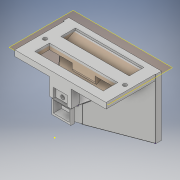
# Autodesk Inventor part: ventilador controladora
Saved by Autodesk Inventor 2019 (Build 230136000, 136)
## iProperties
Created: 2018-08-15
Part Number: ventilador controladora
Material: Genérico
Document SubType Name: Modeling
Designer: Albert Garangou Culebras
Density: 1 g/cm^3
Appearance: Valor por defecto
Author: Albert Garangou Culebras
Autodesk Inventor part; units mm, degrees
sketch "Boceto1" plane through (0, 0, 0) normal (0, 0, 1) x (1, 0, 0)
  line L0 (0, 0) -> (16, 0)
  line L1 (16, 0) -> (16, -12)
  line L2 (16, -12) -> (0, -12)
  line L3 (0, -12) -> (0, 0)
  line L4 (1, -1) -> (15, -1)
  line L5 (15, -1) -> (15, -11)
  line L6 (15, -11) -> (1, -11)
  line L7 (1, -11) -> (1, -1)
  dimension "d0" = 16
  dimension "d1" = 12
  constraints: 16 end point, 4 parallel, 2 horizontal, 2 perpendicular
  measures "d0" distance of L1.end L2.end
  measures "d1" distance of L0.end L1.end
ref_plane "Plano de trabajo3" through (0, 0, -40) normal (0, 0, -1) x (-1, 0, 0)
sketch "Boceto4" plane through (0, 0, -40) normal (0, 0, -1) x (-1, 0, 0)
  line L0 (0, -12) -> (0, 0) projected
  line L1 (0, -6) -> (-16, -6)
  line L2 (-8, -31) -> (-48, -31)
  line L3 (-8, -31) -> (32, -31)
  line L4 (32, -31) -> (32, 19)
  line L5 (32, 19) -> (-48, 19)
  line L6 (-48, 19) -> (-48, -31)
  dimension "d8" = 40
  dimension "d9" = 40
  dimension "d10" = 80
  constraints: 12 end point, 2 horizontal, 1 midpoint, 1 perpendicular, 1 vertical
  measures "d8" distance of L2.start L2.end
  measures "d9" distance of L2.start L3.end
  measures "d10" distance of L4.end L5.end
extrude "Extrusión2" add sketch "Boceto1" against normal blind 40
loft "Solevación1" add profiles "Boceto4" section 1 edges at (1, -6, 0) (8, -1, 0) (15, -6, 0) (8, -11, 0)
sketch "Boceto5" plane through (0, 0, -40) normal (0, 0, -1) x (-1, 0, 0)
  line L0 (30, -29) -> (-46, -29)
  line L1 (-46, -29) -> (-46, 17)
  line L2 (-46, 17) -> (30, 17)
  line L3 (30, 17) -> (30, -29)
  point P0 (0, 0)
  constraints: 8 end point, 2 parallel, 1 horizontal, 1 perpendicular
sketch "Boceto6" plane through (0, 0, 0) normal (0, 0, 1) x (1, 0, 0)
  line L0 (1, -11) -> (15, -11)
  line L1 (15, -11) -> (15, -1)
  line L2 (15, -1) -> (1, -1)
  line L3 (1, -1) -> (1, -11)
  point P0 (0, 0)
  constraints: 8 end point, 2 parallel, 1 horizontal, 1 perpendicular
loft "Solevación2" cut profiles "Boceto6", "Boceto5"
sketch "Boceto7" plane through (0, 0, 0) normal (0, 0, 1) x (1, 0, 0)
  line L0 (0, 0) -> (16, 0) projected
  line L1 (16, -12) -> (0, -12) projected
  line L2 (0, 0) -> (16, 0)
  line L3 (16, 0) -> (16, -12)
  line L4 (16, -12) -> (0, -12)
  line L5 (0, -12) -> (0, 0)
  line L6 (1, -11) -> (1, -1) projected
  line L7 (1, -1) -> (15, -1)
  line L8 (15, -1) -> (15, -11)
  line L9 (15, -11) -> (1, -11)
  line L10 (1, -11) -> (1, -1)
  constraints: 16 end point, 4 parallel, 2 horizontal, 2 perpendicular
extrude "Extrusión3" add sketch "Boceto7" against normal blind 5
sketch "Boceto8" plane through (0, 0, 0) normal (0, 0, 1) x (1, 0, 0)
  line L0 (0, 0) -> (16, 0)
  line L1 (16, 0) -> (16, -12)
  line L2 (16, -12) -> (0, -12)
  line L3 (0, -12) -> (0, 0)
  line L4 (15, -1) -> (15, -11) projected
  line L5 (1, -1) -> (15, -1)
  line L6 (15, -1) -> (15, -11)
  line L7 (15, -11) -> (1, -11)
  line L8 (1, -11) -> (1, -1)
  constraints: 16 end point, 4 parallel, 2 horizontal, 2 perpendicular
extrude "Extrusión4" add sketch "Boceto8" along normal blind 3
ref_plane "Plano de trabajo7" through (-19.527001, -29, -48.116575) normal (0.7904151, 0, -0.6125717) x (-0.6125717, 0, -0.7904151)
sketch "Boceto17" plane through (-19.527001, -29, -48.116575) normal (0.7904151, 0, -0.6125717) x (-0.6125717, 0, -0.7904151)
  line L0 (-46.555447, 46) -> (0, 46)
  line L1 (-10.291798, 46) -> (-10.291798, 0)
  line L2 (-10.291798, 0) -> (-38.576069, 10)
  line L3 (-38.576069, 10) -> (-38, 37)
  line L4 (-38, 37) -> (-10.291798, 46)
  point P0 (-49.993752, 29)
  dimension "d37" = 30
  constraints: 8 end point, 1 point on line, 1 vertical
  measures "d37" distance of L1.end L2.end
ref_plane "Plano de trabajo8" through (35.724604, -29, -47.963432) normal (-0.7904151, 0, -0.6125717) x (-0.6125717, 0, 0.7904151)
sketch "Boceto18" plane through (35.724604, -29, -47.963432) normal (-0.7904151, 0, -0.6125717) x (-0.6125717, 0, 0.7904151)
  line L0 (0, 46) -> (46.555447, 46)
  line L1 (10.079184, 46) -> (10.079184, 0)
  line L2 (46.555447, 0) -> (0, 0)
  line L3 (10.079184, 0) -> (38.363455, 10)
  line L4 (38.363455, 10) -> (38.363455, 36)
  line L5 (38.363455, 36) -> (10.079184, 46)
  point P0 (59.794899, 29)
  dimension "d39" = 30
  constraints: 8 end point, 2 point on line, 2 vertical
  measures "d39" distance of L1.end L3.end
extrude "Extrusión9" add sketch "Boceto18" along normal blind 0.8
extrude "Extrusión10" add sketch "Boceto17" along normal blind 0.8
ref_plane "Plano de trabajo9" through (0, 19, -2) normal (0, 1, 0) x (1, 0, 0)
sketch "Boceto22" plane through (0, 19, -2) normal (0, 1, 0) x (1, 0, 0)
  line L0 (-13.199031, 38) -> (-30, 38)
  line L1 (-30, 38) -> (13, 38) construction
  line L2 (16, -0.787879) -> (48, 38)
  line L3 (48, 38) -> (48, -5)
  line L4 (48, 38) -> (91, 38) construction
  line L5 (48, -5) -> (-31.751276, -5)
  line L6 (48, 38) -> (-32, 38)
  line L7 (-31.751276, 38) -> (-31.751276, -5)
  line L8 (-31.751276, 38) -> (11.248724, 38) construction
  line L9 (-31.751276, -5) -> (-21.751276, -5)
  line L10 (-21.751276, -5) -> (-21.751276, 38)
  line L11 (-21.751276, 38) -> (-31.751276, 38)
  line L12 (48, -5) -> (38, -5)
  line L13 (38, -5) -> (38, 38)
  line L14 (48, 38) -> (38, 38)
  point P0 (0, -2)
  dimension "d46" = 90
  dimension "d47" = 43
  dimension "d49" = 90
  dimension "d50" = 10
  dimension "d51" = 43
  dimension "d52" = 90
  dimension "d53" = 10
  dimension "d54" = 43
  constraints: 24 end point, 4 perpendicular, 4 point on line, 3 horizontal, 1 collinear
  measures "d46" angle of L3 L4
  measures "d47" distance of L2.end L3.end
  measures "d49" angle of L7 L8
  measures "d50" distance of L5.end L9.end
  measures "d51" distance of L9.end L10.end
  measures "d52" angle of L10 L9
  measures "d53" distance of L3.end L12.end
  measures "d54" distance of L12.end L13.end
extrude "Extrusión11" add sketch "Boceto22" against normal blind 3 contours L10 L5 L7 L6 L0 | L6 L2 L13 | L3 L5 L13 L2
sketch "Boceto24" plane through (38, 19, -40) normal (-1, 0, 0) x (0, 0, 1)
  line L0 (0, 0) -> (43, 0) projected
  line L1 (35.5, -2) -> (35.5, 0)
  line L2 (35.5, 0) -> (43, 0)
  line L3 (43, 0) -> (43, -2)
  line L4 (35.5, -2) -> (35.5, -3)
  line L5 (43, -3) -> (6, -3) projected
  line L6 (43, -3) -> (35.5, -3)
  line L7 (43, -3) -> (43, -2)
  line L8 (43, 0) -> (43, -3) projected
  point P0 (40, -19)
  dimension "d57" = 7.5
  constraints: 12 end point, 2 collinear, 2 point on line, 1 parallel, 1 vertical
  measures "d57" distance of L1.end L2.end
extrude "Extrusión12" add sketch "Boceto24" along normal blind 60
sketch "Boceto25" plane through (-31.751276, 19, 3) normal (0, 0, 1) x (1, 0, 0)
  line L0 (79.751276, -3) -> (0, -3)
  line L1 (39.875638, -3) -> (49.375638, -3)
  line L2 (39.875638, -3) -> (30.375638, -3)
  line L3 (30.375638, -3) -> (30.375638, -19)
  line L4 (30.375638, -19) -> (49.375638, -19)
  line L5 (49.375638, -19) -> (49.375638, -3)
  point P0 (31.751276, -19)
  dimension "d60" = 9.5
  dimension "d61" = 9.5
  dimension "d63" = 16
  dimension "d64" = 19
  constraints: 10 end point, 2 perpendicular, 2 point on line, 1 midpoint
  measures "d60" distance of L1.start L1.end
  measures "d61" distance of L1.start L2.end
  measures "d63" distance of L2.end L3.end
  measures "d64" distance of L3.end L4.end
extrude "Extrusión13" add sketch "Boceto25" against normal blind 7.5
sketch "Boceto27" plane through (0, 0, -40) normal (0, 0, -1) x (-1, 0, 0)
  line L0 (31.751276, 19) -> (-48, 19)
  line L1 (31.751276, 19) -> (-48, 19)
  line L2 (-48, 19) -> (-48, -31)
  line L3 (-48, -31) -> (31.751276, -31)
  line L4 (31.751276, -31) -> (31.751276, 19)
  line L5 (30, 16) -> (30, -29)
  line L6 (-46, -29) -> (-46, 16)
  line L7 (30, 17) -> (-46, 17)
  line L8 (-46, 17) -> (-46, -29)
  line L9 (-46, -29) -> (30, -29)
  line L10 (30, -29) -> (30, 17)
  point P0 (0, 0)
  constraints: 16 end point, 4 parallel, 2 horizontal, 2 perpendicular
extrude "Extrusión15" add sketch "Boceto27" along normal blind 5
sketch "Boceto28" plane through (0, -12, -2) normal (0, -1, 0) x (1, 0, 0)
  line L0 (16, 1) -> (0, 1)
  line L1 (0, 1) -> (0, 5)
  line L2 (0, 5) -> (16, 5)
  line L3 (16, 5) -> (16, 1)
  point P0 (0, 2)
  constraints: 8 end point, 2 parallel, 1 horizontal, 1 perpendicular
extrude "Extrusión16" add sketch "Boceto28" against normal blind 12
sketch "Boceto30" plane through (0, 0, 3) normal (0, 0, 1) x (1, 0, 0)
  line L0 (15, -11) -> (1, -11)
  line L1 (1, -11) -> (1, -1)
  line L2 (1, -1) -> (15, -1)
  line L3 (15, -1) -> (15, -11)
  point P0 (0, 0)
  constraints: 8 end point, 2 parallel, 1 horizontal, 1 perpendicular
extrude "Extrusión17" cut sketch "Boceto30" against normal blind 7.75
sketch "Boceto31" plane through (-32, -31, -40) normal (-0.7713733, 0, 0.636383) x (0.636383, 0, 0.7713733)
  line L0 (50.223865, 30.580645) -> (50.223865, 19.419355)
  line L1 (50.223865, 30.580645) -> (50.223865, 19.419355)
  line L2 (50.223865, 19.419355) -> (36, 14)
  line L3 (36, 14) -> (36, 36.115281)
  line L4 (50.284188, 30.606061) -> (7.778335, 47)
  line L5 (50.223865, 30.580645) -> (36, 36.115281)
  point P0 (51.219186, 31)
  constraints: 8 end point, 1 collinear, 1 parallel, 1 point on line
extrude "Extrusión18" add sketch "Boceto31" against normal blind 1
sketch "Boceto32" plane through (16, -11.606061, -1.212121) normal (0.7713733, 0, 0.636383) x (0.636383, 0, -0.7713733)
  line L0 (0.060322, 11.186706) -> (0.779165, 11.606061)
  line L1 (0.060322, -0.000081) -> (0.060322, 11.186706)
  line L2 (0.060322, 11.186706) -> (9.130626, 14.733682)
  line L3 (0, 11.212121) -> (42.505852, 27.606061)
  line L4 (9.130626, -0.000163) -> (9.130626, 14.733682)
  line L5 (-0.626449, 30.606061) -> (-0.626449, -19.393939)
  line L6 (9.130626, -0.000163) -> (9.130626, -3.535488)
  line L7 (9.130626, -3.535488) -> (0.060322, -0.000325)
  line L8 (0.060322, 0.025415) -> (0.060322, 11.186706)
  line L9 (0.060322, -0.000325) -> (0.060322, 11.186706)
  point P0 (-11.117125, 11.606061)
  constraints: 12 end point, 2 vertical, 1 collinear, 1 parallel, 1 point on line
extrude "Extrusión19" add sketch "Boceto32" against normal blind 1 contours L2 L4 L6 L7 L1
sketch "Boceto33" plane through (0, -12, -2) normal (0, -0.8944272, 0.4472136) x (1, 0, 0)
  line L0 (0, -0.700786) -> (0, 4.665778)
  line L1 (0, 0.854238) -> (-9.541728, -11.818024)
  line L2 (-8.31884, -11.8619) -> (-4.377414, -6.627335)
  line L3 (-9.541728, -11.818024) -> (25.370549, -11.818024)
  line L4 (11.591907, -17.557996) -> (11.591907, -5.930443)
  line L5 (16, 0.880875) -> (19.630054, -4.038548)
  line L6 (25.370549, -11.818024) -> (16, 0.880875)
  line L7 (16, 4.472136) -> (16, 0)
  line L8 (16, 0.880875) -> (16, 0)
  line L9 (16, 0) -> (0, 0)
  line L10 (0, 0) -> (0, 0.854238)
  line L11 (0, 4.472136) -> (0, 0)
  point P0 (0, 7.155418)
  point P1 (0, 0.09651)
  point P2 (0, 5.275946)
  constraints: 12 end point, 3 point on line, 2 collinear, 1 parallel, 1 perpendicular
extrude "Extrusión20" add sketch "Boceto33" against normal blind 1
sketch "Boceto34" plane through (0, 0, -2) normal (0, 0.8944272, 0.4472136) x (1, 0, 0)
  line L0 (30.35, 18.56614) -> (-13.525, 17.448106)
  line L1 (0, -0.880875) -> (-27.05, 35.777088)
  line L2 (-13.525, 17.448106) -> (0.825, -1.998909)
  line L3 (0.825, -1.998909) -> (0, -0.036399)
  line L4 (0, 0) -> (0, -0.880875)
  line L5 (0, 0) -> (16, 0)
  line L6 (16, 0) -> (0, 0)
  line L7 (16, -0.880875) -> (16, 0)
  line L8 (16, 0) -> (16, -0.880875)
  line L9 (16, -0.880875) -> (30.35, 18.56614)
  line L10 (16, -0.880875) -> (43.05, 35.777088)
  point P0 (0, -1.788854)
  point P1 (17.624362, 2.236068)
  point P2 (17.624362, 2.795085)
  constraints: 12 end point, 2 collinear, 1 midpoint, 2 other
extrude "Extrusión21" [suppressed]
sketch "Boceto35" plane through (16, -11.606061, -1.212121) normal (0.7713733, 0, 0.636383) x (0.636383, 0, -0.7713733)
  line L0 (0, 0) -> (16, -6.170986)
  line L1 (9.130626, -3.52156) -> (50.284188, -19.393939)
  line L2 (16, -6.170986) -> (16, 17.383107)
  line L3 (0, 11.212121) -> (42.505852, 27.606061)
  line L4 (0, 0) -> (0, 11.212121)
  line L5 (0, 11.212121) -> (16, 17.383107)
  line L6 (0, 11.212121) -> (0.607749, 11.606061)
  line L7 (0, 11.212121) -> (0, 0)
  line L8 (1.212121, 11.606061) -> (1.212121, 0.332344)
  point P0 (-11.117125, 11.606061)
  point P1 (1.212121, 10.879778)
  point P2 (1.212121, 0.332344)
  point P3 (0.30303, 10.426431)
  point P4 (0.30303, 0.78569)
  constraints: 8 end point, 2 point on line, 2 vertical, 1 other
extrude "Extrusión22" add sketch "Boceto35" against normal blind 1
sketch "Boceto37" plane through (0, 0, 3) normal (0, 0, 1) x (1, 0, 0)
  line L0 (0, -12) -> (16, -12) projected
  line L1 (0, -12) -> (16, -12)
  line L2 (16, -12) -> (16, 0)
  line L3 (16, 0) -> (0, 0)
  line L4 (0, 0) -> (0, -12)
  line L5 (1, -1) -> (15, -1) projected
  line L6 (15, -1) -> (1, -1)
  line L7 (1, -1) -> (1, -11)
  line L8 (1, -11) -> (15, -11)
  line L9 (15, -11) -> (15, -1)
  constraints: 16 end point, 4 parallel, 2 horizontal, 2 perpendicular
extrude "Extrusión23" cut sketch "Boceto37" against normal blind 1
sketch "Boceto38" plane through (-31.751276, 19, 3) normal (0, 0, 1) x (1, 0, 0)
  line L0 (30.375638, -17.75) -> (49.375638, -17.75)
  line L1 (30.375638, -19) -> (49.375638, -19)
  line L2 (39.875638, -19) -> (39.875638, -14)
  line L3 (39.875638, -14) -> (39.875638, -15)
  circle A0 centre (39.875638, -15) radius 1.75
  point P0 (31.751276, -19)
  dimension "d94" = 5
  dimension "d146" = 1
  dimension "d147" = 3.5
  constraints: 4 end point, 2 coincident, 1 centre point, 1 midpoint, 1 point on line
  measures "d94" distance of L2.start L2.end
  measures "d146" distance of L3.start L3.end
  measures "d147" diameter of A0
extrude "Extrusión24" cut sketch "Boceto38" against normal blind 7.75
sketch "Boceto39" plane through (-31.751276, 19, 3) normal (0, 0, 1) x (1, 0, 0)
  line L0 (34.424818, -19) -> (45.424818, -19)
  line L1 (45.424818, -9.5) -> (45.674818, -9.5)
  line L2 (45.674818, -9.5) -> (45.674818, -19)
  line L3 (16.800456, -9.5) -> (16.550456, -9.5)
  line L4 (45.674818, -19) -> (33.674818, -19)
  line L5 (45.424818, -9.5) -> (33.674818, -9.5)
  line L6 (33.674818, -19) -> (33.674818, -9.5)
  line L7 (30.375638, -17.75) -> (49.375638, -17.75)
  point P0 (30.375638, -3)
  point P1 (49.375638, -3)
  point P2 (16.550456, -19)
  dimension "d100" = 9.5
  dimension "d103" = 0.25
  dimension "d104" = 0.25
  dimension "d109" = 12
  constraints: 14 end point, 2 perpendicular, 1 horizontal
  measures "d100" distance of L0.end L1.start
  measures "d103" distance of L1.start L1.end
  measures "d104" distance of L3.start L3.end
  measures "d109" distance of L2.end L4.end
extrude "Extrusión25" cut sketch "Boceto39" against normal blind 2
sketch "Boceto40" plane through (0, 16, -2) normal (0, -1, 0) x (1, 0, 0)
  line L0 (-31.751276, -38) -> (-31.751276, 5)
  line L1 (-31.751276, 5) -> (-31.751276, -38)
  line L2 (-31.751276, -16.5) -> (-22, -16.5)
  circle A0 centre (-26.875638, -16.5) radius 1.65
  circle A1 centre (43, -16.5) radius 1.65
  point P0 (0, 2)
  dimension "d105" = 3.3
  dimension "d106" = 3.3
  constraints: 4 end point, 2 centre point, 2 midpoint, 1 collinear, 1 horizontal
  measures "d105" diameter of A0
  measures "d106" diameter of A1
extrude "Extrusión26" cut sketch "Boceto40" against normal blind 38.5
sketch "Boceto41" plane through (0, 16, -2) normal (0, -1, 0) x (1, 0, 0)
  line L0 (38, -35.777778) -> (38, -38)
  line L1 (38, -35.777778) -> (38, -38)
  line L2 (38, -38) -> (46, -38)
  line L3 (38, -38) -> (46, -38)
  line L4 (46, -38) -> (44.288464, -35.777778)
  line L5 (44.288464, -35.777778) -> (38, -35.777778)
  line L6 (-21.751276, -2.5) -> (-21.751276, -38)
  line L7 (-21.751276, -35.777778) -> (-21.751276, -38)
  line L8 (-30, -38) -> (-21.751276, -38)
  line L9 (-21.751276, -38) -> (-30, -38)
  line L10 (-30, -38) -> (-28.277778, -35.777778)
  line L11 (-30, -38) -> (-28.277778, -35.777778)
  line L12 (-28.277778, -35.777778) -> (-21.751276, -35.777778)
  line L13 (-28.277778, -35.777778) -> (-21.751276, -35.777778)
  point P0 (0, 2)
  constraints: 16 end point, 4 collinear, 2 parallel, 1 perpendicular, 1 point on line
extrude "Extrusión27" cut sketch "Boceto41" against normal blind 1
sketch "Boceto42" plane through (38, 16, -37.777778) normal (1, 0, 0) x (0, 0, -1)
  line L0 (2.222222, 1) -> (0, 1)
  line L1 (0, 0) -> (0, 1)
  line L2 (2.222222, 1) -> (0, 0)
  line L3 (0, 0) -> (0, 1)
  line L4 (0, 1) -> (2.222222, 1)
  point P0 (-37.777778, -16)
  constraints: 6 end point, 1 collinear, 1 perpendicular
sketch "Boceto43" plane through (-21.751276, 16, -37.777778) normal (-1, 0, 0) x (0, 0, 1)
  line L0 (0, 0) -> (-2.222222, 1)
  line L1 (-2.222222, 1) -> (0, 0)
  line L2 (0, 0) -> (0, 1)
  line L3 (0, 0) -> (0, 1)
  line L4 (0, 1) -> (-2.222222, 1)
  point P0 (37.777778, -16)
  constraints: 6 end point, 2 collinear, 1 perpendicular
extrude "Extrusión29" add sketch "Boceto43" along normal blind 8.75
extrude "Extrusión30" add sketch "Boceto42" along normal blind 8.25
sketch "Boceto44" plane through (0, 0, 3) normal (0, 0, 1) x (1, 0, 0)
  line L0 (13.923542, 0) -> (17.624362, 0)
  line L1 (17.624362, 0) -> (17.624362, 1)
  line L2 (17.624362, 1.25) -> (17.624362, 0.590523)
  line L3 (17.624362, 1.025) -> (-1.375638, 1.025)
  line L4 (17.624362, 1) -> (-1.375638, 1.025)
  line L5 (-1.375638, 1.025) -> (-1.376954, 0.025002)
  line L6 (-1.376954, 0.025002) -> (17.624362, 0)
  point P0 (0, 0)
  dimension "d118" = 1
  constraints: 8 end point, 2 perpendicular, 1 point on line
  measures "d118" distance of L0.end L1.end
extrude "Extrusión31" cut sketch "Boceto44" against normal blind 7.25 contours L6 L5 L4 L1
sketch "Boceto45" plane through (-0.65, 0, -2) normal (0, -1, 0) x (1, 0, 0)
  line L0 (-0.725638, 5) -> (2.573542, 5)
  line L1 (2.573542, 5) -> (-0.725638, 5)
  line L2 (-0.725638, 5) -> (-0.725638, -0.879561)
  line L3 (-0.725638, 5) -> (-0.725638, -0.879561)
  line L4 (0.65, 0) -> (0.65, 0.787879)
  line L5 (-0.725638, -0.879561) -> (0.65, 0)
  line L6 (0.65, 0) -> (0.65, 4)
  line L7 (0.65, 4) -> (2.573542, 4)
  line L8 (2.573542, 4) -> (2.573542, 5)
  line L9 (2.573542, 4) -> (2.573542, 5)
  line L10 (14.573542, 5) -> (18.274362, 5)
  line L11 (14.573542, 5) -> (18.274362, 5)
  line L12 (18.274362, 5) -> (14.573542, 5)
  line L13 (2.573542, 4) -> (14.573542, 4)
  line L14 (14.573542, 5) -> (14.573542, 4)
  line L15 (14.573542, 4) -> (16.65, 4)
  line L16 (16.65, 0.787879) -> (16.65, 0)
  line L17 (16.65, 4) -> (16.65, 0.787879)
  line L18 (18.274362, -1.181045) -> (17.3, 0)
  line L19 (16.65, 0.787879) -> (18.274362, -1.181045)
  line L20 (18.274362, 5) -> (18.274362, -1.181045)
  line L21 (18.274362, -1.181045) -> (18.274362, 5)
  line L22 (18.274362, 5) -> (14.573542, 5)
  point P0 (0.65, 2)
  constraints: 26 end point, 7 perpendicular, 3 collinear, 1 horizontal, 1 parallel
extrude "Extrusión32" cut sketch "Boceto45" against normal blind 0.5
sketch "Boceto46" plane through (-21.751276, 19, -4.5) normal (1, 0, 0) x (0, 0, -1)
  line L0 (35.5, 0) -> (29.5, -3)
  line L1 (0, 0) -> (35.5, 0)
  line L2 (35.5, 0) -> (0, 0)
  line L3 (17.75, 0) -> (22.75, 0)
  line L4 (22.75, 0) -> (12.75, 0)
  line L5 (22.75, 0) -> (22.75, -3)
  line L6 (-7.5, -3) -> (35.198516, -3)
  line L7 (22.75, -3) -> (12.75, -3)
  line L8 (15.65, -3) -> (12.35, -3)
  line L9 (29.5, -3) -> (0, -3)
  line L10 (12.75, -3) -> (12.75, 0)
  point P0 (-4.5, -19)
  dimension "d123" = 5
  dimension "d124" = 10
  constraints: 12 end point, 4 point on line, 1 collinear, 1 midpoint, 1 perpendicular, 1 vertical
  measures "d123" distance of L3.start L3.end
  measures "d124" distance of L3.end L4.end
extrude "Extrusión33" add sketch "Boceto46" along normal blind 61.5 contours L5 L6 L10 L1
sketch "Boceto47" plane through (0, 16, -2) normal (0, -1, 0) x (1, 0, 0)
  line L0 (38, -15.25) -> (38, -2.5)
  line L1 (-21.751276, -15.25) -> (38, -15.25)
  line L2 (38, -15.25) -> (-21.751276, -15.25)
  line L3 (-21.751276, -32) -> (-21.751276, -25.25)
  line L4 (-21.751276, -15.25) -> (-21.751276, -25.25)
  line L5 (-21.751276, -25.25) -> (38, -25.25)
  line L6 (-21.751276, -25.25) -> (38, -25.25)
  line L7 (38, -25.25) -> (38, -15.25)
  line L8 (-21.751276, -15.25) -> (-21.751276, -2.5)
  line L9 (-21.751276, -15.25) -> (-21.751276, -25.25)
  line L10 (8.124362, -15.25) -> (-1.875638, -15.25)
  line L11 (-1.875638, -15.25) -> (18.124362, -15.25)
  line L12 (18.124362, -15.25) -> (18.124362, -25.25)
  line L13 (-1.875638, -15.25) -> (-1.875638, -25.25)
  line L14 (18.124362, -25.25) -> (-1.875638, -25.25)
  point P0 (0, 2)
  dimension "d127" = 10
  dimension "d128" = 20
  constraints: 20 end point, 5 perpendicular, 4 point on line, 3 collinear, 1 midpoint
  measures "d127" distance of L10.start L10.end
  measures "d128" distance of L10.end L11.end
extrude "Extrusión34" add sketch "Boceto47" along normal blind 4.5 contours L1 L12 L5 L13
sketch "Boceto48" plane through (-21.751276, 19, -40) normal (0, 0.8944272, 0.4472136) x (1, 0, 0)
  line L0 (19.875638, -23.702321) -> (19.875638, -16.77051)
  line L1 (19.875638, -23.702321) -> (39.875638, -23.702321)
  line L2 (39.875638, -23.702321) -> (39.875638, -14.702321)
  line L3 (39.875638, -14.702321) -> (19.875638, -14.702321)
  line L4 (19.875638, -16.77051) -> (19.875638, -14.254933)
  line L5 (39.875638, -14.702321) -> (19.875638, -14.702321)
  point P0 (21.751276, -44.274146)
  dimension "d131" = 9
  constraints: 8 end point, 2 perpendicular, 1 collinear, 1 horizontal, 1 point on line
  measures "d131" distance of L1.end L2.end
extrude "Extrusión35" add sketch "Boceto48" along normal blind 7.25
sketch "Boceto49" plane through (0, 16, -2) normal (0, -1, 0) x (1, 0, 0)
  line L0 (-21.751276, -15.25) -> (-21.751276, -2.5)
  line L1 (-21.751276, -15.25) -> (-21.751276, -2.5)
  line L2 (38, -2.5) -> (17.624362, -2.5)
  line L3 (-21.751276, -2.5) -> (38, -2.5)
  line L4 (38, -2.5) -> (38, -15.25)
  line L5 (38, -2.5) -> (38, -15.25)
  line L6 (-21.751276, -15.25) -> (-1.875638, -15.25)
  line L7 (38, -15.25) -> (-21.751276, -15.25)
  point P0 (0, 2)
  constraints: 8 end point, 2 collinear, 1 perpendicular
extrude "Extrusión36" cut sketch "Boceto49" along normal blind 5.25
sketch "Boceto50" plane through (0, 19, -2) normal (0, 1, 0) x (1, 0, 0)
  line L0 (48, -5) -> (48, 43)
  line L1 (-31.751276, 43) -> (48, 43)
  line L2 (48, -5) -> (-31.751276, -5)
  line L3 (-31.751276, -5) -> (-31.751276, 43)
  line L4 (-31.751276, 43) -> (48, 43)
  line L5 (48, 43) -> (48, -5)
  line L6 (38, 2.5) -> (38, 15.25)
  line L7 (-21.751276, 15.25) -> (-21.751276, 2.5)
  line L8 (38, 2.5) -> (-21.751276, 2.5)
  line L9 (-21.751276, 2.5) -> (-21.751276, 15.25)
  line L10 (-21.751276, 15.25) -> (38, 15.25)
  line L11 (38, 15.25) -> (38, 2.5)
  line L12 (18.124362, 25.25) -> (38, 25.25)
  line L13 (-21.751276, 25.25) -> (-21.751276, 38)
  line L14 (38, 25.25) -> (-21.751276, 25.25)
  line L15 (-21.751276, 25.25) -> (-21.751276, 38)
  line L16 (-21.751276, 38) -> (38, 38)
  line L17 (38, 38) -> (38, 25.25)
  circle A0 centre (43, 16.5) radius 1.65
  circle A1 centre (43, 16.5) radius 1.65
  circle A2 centre (-26.875638, 16.5) radius 1.65
  circle A3 centre (-26.875638, 16.5) radius 1.65
  point P0 (0, -2)
  constraints: 24 end point, 6 parallel, 3 horizontal, 3 perpendicular, 2 centre point, 2 coincident
extrude "Extrusión37" add sketch "Boceto50" along normal blind 2
sketch "Boceto51" plane through (0, 0, 2) normal (0, 0, 1) x (1, 0, 0)
  line L0 (15, -0.488405) -> (0, -0.488405)
  line L1 (0, -0.488405) -> (0, 0.453578)
  line L2 (0, -12) -> (0, 0.02319)
  line L3 (0, 0.453578) -> (16.256322, 0.453578)
  line L4 (16.256322, 0.453578) -> (16.256322, -0.488405)
  line L5 (16.256322, -0.488405) -> (15, -0.488405)
  point P0 (0, 0)
  point P1 (0, -0.419355)
  point P2 (16, 0)
  point P3 (16, -0.393939)
  constraints: 10 end point, 2 collinear, 2 perpendicular, 1 horizontal, 1 point on line
extrude "Extrusión38" cut sketch "Boceto51" against normal blind 3.25
sketch "Boceto52" plane through (16, -12, 2) normal (1, 0, 0) x (0, 0, -1)
  line L0 (0, 0) -> (0, 11.511595)
  line L1 (0, 0) -> (0, 11.511595)
  line L2 (3.212121, 11.511595) -> (0, 11.511595)
  line L3 (0, 11.511595) -> (3.212121, 11.511595)
  line L4 (3.212121, 11.511595) -> (3.212121, 0)
  line L5 (3.212121, 11.511595) -> (3.212121, 0.393939)
  line L6 (0, 0) -> (4, 0)
  line L7 (3.212121, 0) -> (0, 0)
  point P0 (2, 12)
  constraints: 8 end point, 3 collinear, 1 vertical
extrude "Extrusión39" add sketch "Boceto52" along normal blind 0.3
sketch "Boceto53" plane through (0, -12, -2) normal (-1, 0, 0) x (0, 0, 1)
  line L0 (4, 11.511595) -> (0.787879, 11.511595)
  line L1 (4, 11.511595) -> (0.787879, 11.511595)
  line L2 (0.787879, 11.511595) -> (0.787879, 0)
  line L3 (4, 0) -> (0, 0)
  line L4 (0.787879, 0) -> (4, 0)
  line L5 (4, 0) -> (4, 11.511595)
  point P0 (2, 12)
  constraints: 8 end point, 2 collinear, 2 perpendicular
extrude "Extrusión40" add sketch "Boceto53" along normal blind 0.3
sketch "Boceto54" plane through (0, -12, -2) normal (0, -1, 0) x (1, 0, 0)
  line L0 (16, 0.787879) -> (16.3, 0.787879)
  line L1 (16.3, 4) -> (16.3, 0.787879)
  line L2 (16.3, 0.787879) -> (16.3, 4)
  line L3 (16.3, 4) -> (-0.3, 4)
  line L4 (16.3, 4) -> (-0.3, 4)
  line L5 (-0.3, 0.787879) -> (-0.3, 4)
  line L6 (-0.3, 4) -> (-0.3, 0.787879)
  line L7 (-0.3, 0.787879) -> (16.3, 0.787879)
  point P0 (0, 2)
  constraints: 8 end point, 2 collinear, 2 perpendicular
extrude "Extrusión41" add sketch "Boceto54" along normal blind 0.75
sketch "Boceto55" plane through (48, -31, -40) normal (0.7713733, 0, 0.636383) x (0.636383, 0, -0.7713733)
  line L0 (0, 0) -> (0, 47)
  line L1 (0, 47) -> (0, 0)
  line L2 (-49.676439, 19) -> (-50.284188, 19.393939)
  line L3 (0, 0) -> (-50.284188, 19.393939)
  line L4 (-47.731696, 31.590523) -> (-7.778335, 47)
  line L5 (-50.284188, 30.511595) -> (-7.778335, 47)
  line L6 (-7.778335, 47) -> (0, 47)
  line L7 (-1.272766, 48) -> (2.5841, 48)
  line L8 (-50.284188, 19.393939) -> (-44.57999, 17.193907)
  line L9 (-50.284188, 19.393939) -> (-45.619136, 17.594691)
  line L10 (-45.619136, 17.594691) -> (-45.08732, 17.389577)
  line L11 (-45.08732, 17.389577) -> (-45.08732, 32.527507)
  point P0 (-61.401313, 31)
  point P1 (-45.619136, 32.321211)
  dimension "d159" = 5
  dimension "d160" = 0.57
  constraints: 14 end point, 4 point on line, 1 collinear, 1 parallel, 1 vertical
  measures "d159" distance of L2.end L9.end
  measures "d160" distance of L9.end L10.end
extrude "Extrusión42" add sketch "Boceto55" along normal blind 0.4
sketch "Boceto56" plane through (-32, -31, -40) normal (-0.7713733, 0, 0.636383) x (0.636383, 0, 0.7713733)
  line L0 (50.284188, 19.393939) -> (49.676439, 19)
  line L1 (50.093273, 30.511595) -> (8.041918, 47)
  line L2 (7.778335, 47) -> (0.390841, 47)
  line L3 (8.041918, 47) -> (0.390841, 47)
  line L4 (0.390841, 47) -> (0.390841, 50)
  line L5 (0.390841, 49.849258) -> (0, 50)
  line L6 (0.390841, 50) -> (0, 50)
  line L7 (35.559487, 13.714819) -> (0, 0)
  line L8 (0, 50) -> (0, 0)
  line L9 (0, 0) -> (50.284188, 19.393939)
  line L10 (60.456983, 30.511595) -> (50.254969, 30.511595)
  line L11 (50.093273, 30.511595) -> (45.43832, 32.33681)
  line L12 (45.43832, 17.524953) -> (45.201514, 17.444807)
  line L13 (48.73986, 18.798313) -> (35.450552, 13.714819)
  line L14 (45.201514, 17.444807) -> (44.968015, 17.355487)
  line L15 (44.968015, 17.355487) -> (45.108115, 17.409079)
  line L16 (45.108115, 17.409079) -> (45.108115, 32.466284)
  point P0 (51.219186, 31)
  point P1 (59.443155, 30.511595)
  point P2 (45.201514, 32.429661)
  dimension "d155" = 5
  dimension "d156" = 0.25
  dimension "d157" = 0.25
  dimension "d158" = 0.15
  constraints: 22 end point, 10 point on line, 3 perpendicular, 1 collinear, 1 vertical
  measures "d155" distance of L11.start L11.end
  measures "d156" distance of L12.start L12.end
  measures "d157" distance of L12.end L14.end
  measures "d158" distance of L14.end L15.end
extrude "Extrusión43" add sketch "Boceto56" along normal blind 0.4 contours L16 L13 L12 L9 L7 L8 L5 L4 L2 L3 L1
sketch "Boceto57" plane through (0, -12, -2) normal (0, -0.8944272, 0.4472136) x (1, 0, 0)
  line L0 (-31.751276, -42.485292) -> (48, -42.485292)
  line L1 (-31.751276, -42.485292) -> (-31.751276, -46.957428)
  line L2 (48, -42.485292) -> (-31.751276, -42.485292)
  line L3 (-31.751276, -42.485292) -> (-32, -42.485292)
  line L4 (-32, -42.485292) -> (-32.308549, -42.257612)
  line L5 (-32, -42.485292) -> (-1.387902, -1)
  line L6 (-3.083828, -3.298306) -> (-32, -42.485292)
  line L7 (-0.340004, 0.420104) -> (-3.308764, -3.603137)
  line L8 (-3.308764, -3.603137) -> (19.308764, -3.603137)
  line L9 (19.307198, -3.601015) -> (19.630054, -4.038548)
  line L10 (48, -42.485292) -> (48, -21.466253)
  line L11 (19.308764, -3.603137) -> (48, -42.485292)
  point P0 (0, 7.155418)
  point P1 (0, 0.880875)
  point P2 (16, 0.880875)
  point P3 (18.968759, -3.142366)
  dimension "d152" = 5
  constraints: 12 end point, 4 point on line, 2 horizontal, 1 perpendicular
  measures "d152" distance of L7.start L7.end
extrude "Extrusión44" add sketch "Boceto57" along normal blind 0.4
sketch "Boceto58" plane through (0, 0, -40) normal (0, 0, -1) x (-1, 0, 0)
  line L0 (32.308549, 19) -> (32.308549, -31)
  line L1 (31.751276, 19) -> (31.751276, -31)
  line L2 (32.308549, -31) -> (31.751276, -31)
  line L3 (31.751276, -31) -> (31.751276, 19)
  line L4 (31.751276, 19) -> (32.308549, 19)
  line L5 (32.308549, 19) -> (32.308549, -31)
  point P0 (0, 0)
  constraints: 8 end point, 2 parallel, 1 horizontal, 1 perpendicular
extrude "Extrusión45" add sketch "Boceto58" along normal blind 5
sketch "Boceto59" plane through (48, -31.357771, -39.821115) normal (0, -0.4472136, -0.8944272) x (-1, 0, 0)
  line L0 (0, 0) -> (28.691236, 0)
  line L1 (80.308549, 0.4) -> (80, 0.4)
  line L2 (0, 0) -> (80, 0)
  line L3 (80, 0) -> (80, 0.4)
  line L4 (80, 0.4) -> (0, 0.4)
  line L5 (0, 0.4) -> (0, 0)
  point P0 (48, 10.238699)
  constraints: 8 end point, 2 parallel, 1 horizontal, 1 perpendicular
sketch "Boceto60" plane through (48, -31, -45) normal (1, 0, 0) x (0, 0, -1)
  line L0 (-5, 2) -> (-5, 47) projected
  line L1 (-5, 0) -> (0, 0) projected
  line L2 (-5, 47) -> (0, 47)
  line L3 (0, 47) -> (0, 0)
  line L4 (0, 0) -> (-5, 0)
  line L5 (-5, 0) -> (-5, 47)
  point P0 (-45, 31)
  constraints: 8 end point, 2 parallel, 1 horizontal, 1 perpendicular
extrude "Extrusión46" add sketch "Boceto60" along normal blind 0.4
sketch "Boceto61" plane through (-32.308549, -31, -45) normal (0, -1, 0) x (1, 0, 0)
  point P0 (32.308549, 45)
sketch "Boceto62" plane through (-32.308549, -31, -39.745447) normal (0.2290022, -0.9330103, 0.2775784) x (0.7713733, 0, -0.636383)
  line L0 (0.28616, 48.321931) -> (0.28616, 0)
  line L1 (0.28616, 48.321931) -> (0, 48)
  line L2 (0, 53.769316) -> (0, 24.416124)
  line L3 (0, 17.992481) -> (0, 0)
  line L4 (0, 48) -> (0, 0)
  line L5 (0, 0) -> (0.28616, 0)
  line L6 (0.4, 0) -> (0, 0)
  line L7 (0.28616, 0) -> (61.996023, 47.500149)
  line L8 (0.28616, 48.321931) -> (0.28616, 0)
  line L9 (0.28616, 0) -> (0, 0)
  point P0 (-0.371373, 58.943367)
  constraints: 10 end point, 2 point on line, 2 vertical, 1 perpendicular
extrude "Extrusión47" add sketch "Boceto62" along normal blind 0.38
sketch "Boceto63" plane through (-32.308549, -31, -45) normal (0, -1, 0) x (1, 0, 0)
  line L0 (0, 5) -> (0, 0)
  line L1 (80.708549, 5) -> (80.708549, 0)
  line L2 (0, 0) -> (80.708549, 0)
  line L3 (80.708549, 0) -> (80.708549, 5)
  line L4 (80.708549, 5) -> (0, 5)
  line L5 (0, 5) -> (0, 0)
  point P0 (32.308549, 45)
  constraints: 8 end point, 2 parallel, 1 horizontal, 1 perpendicular
extrude "Extrusión48" add sketch "Boceto63" along normal blind 0.5
sketch "Boceto64" plane through (-32.308549, 19, -45) normal (-1, 0, 0) x (0, 0, 1)
  line L0 (0, 0) -> (0, -50.5) projected
  line L1 (5, -50.5) -> (0, -50.5) projected
  line L2 (0, 0) -> (5, 0)
  line L3 (5, 0) -> (5, -50.5)
  line L4 (5, -50.5) -> (0, -50.5)
  line L5 (0, -50.5) -> (0, 0)
  point P0 (45, -19)
  constraints: 8 end point, 2 parallel, 1 horizontal, 1 perpendicular
extrude "Extrusión49" add sketch "Boceto64" along normal blind 0.3
sketch "Boceto65" plane through (-32, 19, -40) normal (0, 1, 0) x (1, 0, 0)
  line L0 (-0.608549, 0) -> (-0.608549, 5)
  line L1 (0.248724, 5) -> (0.248724, 0)
  line L2 (-0.608549, 5) -> (0.248724, 5)
  line L3 (0.248724, 5) -> (0.248724, 0)
  line L4 (0.248724, 0) -> (-0.608549, 0)
  line L5 (-0.608549, 0) -> (-0.608549, 5)
  line L6 (80, 0) -> (80, 5)
  line L7 (80.4, 5) -> (80.4, 0)
  line L8 (80, 5) -> (80.4, 5)
  line L9 (80.4, 5) -> (80.4, 0)
  line L10 (80.4, 0) -> (80, 0)
  line L11 (80, 0) -> (80, 5)
  point P0 (32, -40)
  constraints: 16 end point, 4 parallel, 2 horizontal, 2 perpendicular
extrude "Extrusión50" add sketch "Boceto65" along normal blind 2
sketch "Boceto66" plane through (48, 16, -40) normal (0, 1, 0) x (1, 0, 0)
  line L0 (0, 0) -> (0.4, 0) projected
  line L1 (0, 5) -> (0.4, 5)
  line L2 (0.4, 5) -> (0.4, 0)
  line L3 (0.4, 0) -> (0, 0)
  line L4 (0, 0) -> (0, 5)
  point P0 (-48, -40)
  constraints: 8 end point, 2 parallel, 1 horizontal, 1 perpendicular
extrude "Extrusión51" add sketch "Boceto66" along normal blind 3.25
sketch "Boceto67" plane through (-1.375638, 1.25, -4.5) normal (0, 0.8944272, 0.4472136) x (1, 0, 0)
  line L0 (19, -1.474637) -> (19, -1.738726)
  line L1 (19, -1.474637) -> (43.846468, 33.253372)
  line L2 (44.425638, 32.982003) -> (39.375638, 32.982003)
  line L3 (43.846468, 33.253372) -> (39.375638, 32.982003)
  line L4 (39.375638, 39.690207) -> (-20.375638, 39.690207)
  line L5 (39.375638, 32.982003) -> (39.375638, 39.690207)
  line L6 (-20.375638, 39.690207) -> (-20.375638, 40.584634)
  line L7 (39.375638, 39.690207) -> (-20.375638, 39.690207)
  line L8 (-20.375638, 39.690207) -> (-20.375638, 32.982003)
  line L9 (-20.375638, 32.982003) -> (-25.674362, 32.982003)
  line L10 (-20.375638, 32.982003) -> (-25.674362, 32.982003)
  line L11 (-0.000769, -1.810663) -> (-15.421674, 19.087635)
  line L12 (-25.674362, 32.982003) -> (-0.000769, -1.810663)
  line L13 (0, 0) -> (0, 6.596401)
  line L14 (-0.000769, -1.810663) -> (0, 0)
  line L15 (0, 0) -> (18.890828, -0.008027)
  line L16 (18.791749, -0.1423) -> (20.329408, 1.941525)
  line L17 (19, -1.474637) -> (44.425638, 32.982003)
  line L18 (19, -1.474637) -> (18.784666, 0)
  line L19 (0, 0) -> (19, 0)
  point P0 (1.375638, -4.583939)
  constraints: 20 end point, 5 perpendicular, 2 point on line, 1 collinear
extrude "Extrusión52" add sketch "Boceto67" along normal blind 0.5 contours L18 L16 L19 L14 L11 L12 L9 L8 L4 L5 L2 L1 | L1 L2 L17 | L18 L15 L16 | L15 L18 L19 L16
sketch "Boceto68" plane through (-31.751276, 19, -4.5) normal (0, 0, -1) x (-1, 0, 0)
  line L0 (-49.167387, -19) -> (-47.751276, -19)
  line L1 (-49.167387, -19) -> (-49.167387, -17.999726)
  line L2 (-30.375638, -17.975) -> (-49.375638, -18)
  line L3 (-49.375638, -17.975) -> (-30.375638, -17.975)
  line L4 (-30.375638, -19) -> (-30.375638, -17.975)
  line L5 (-30.375638, -17.975) -> (-30.375638, -19)
  line L6 (-49.375638, -19) -> (-30.374322, -18.974998)
  line L7 (-30.375638, -19) -> (-49.167387, -19)
  line L8 (-49.167387, -17.999726) -> (-30.375638, -17.975)
  line L9 (-30.375638, -17.75) -> (-30.374868, -18.559753)
  point P0 (-31.751276, -19)
  constraints: 8 end point, 1 collinear, 1 point on line, 1 vertical, 1 other
extrude "Extrusión53" add sketch "Boceto68" along normal blind 1
sketch "Boceto69" plane through (-1.375638, 0, -5.5) normal (0, -1, 0) x (1, 0, 0)
  line L0 (1.375638, 2.716498) -> (1.375638, 0.5)
  line L1 (1.375638, 0) -> (0, 0)
  line L2 (1.375638, 0) -> (0, 0)
  line L3 (0, 1.049058) -> (0, 0)
  line L4 (0, 0) -> (0, 1.049058)
  line L5 (1.375638, 2.716498) -> (0, 1.049058)
  line L6 (0, 1.049058) -> (1.375638, 2.716498)
  line L7 (1.375638, 2.716498) -> (1.375638, 0.5)
  point P0 (1.375638, 5.5)
  constraints: 8 end point, 2 collinear, 1 horizontal, 1 parallel
sketch "Boceto69 outline for Extrusión54" plane through (-1.375638, 0, -5.5) normal (0, -1, 0) x (1, 0, 0)
  line L0 (1.375638, 0.5) -> (1.375638, 2.716498)
  line L1 (0, 0) -> (1.375638, 0.5)
  line L2 (0, 1.049058) -> (0, 0)
  line L3 (1.375638, 2.716498) -> (0, 1.049058)
extrude "Extrusión54" add sketch "Boceto69 outline for Extrusión54" along normal blind 12.5
sketch "Boceto70" plane through (16, 0, -5) normal (0, -1, 0) x (1, 0, 0)
  line L0 (1.416111, 0.5) -> (0, 2.216498)
  line L1 (0.036755, 2.171947) -> (1.416111, 0.5)
  line L2 (1.416111, 0.5) -> (1.416111, -0.072186)
  line L3 (1.416111, -0.5) -> (0, -0.5)
  line L4 (0, 2.216498) -> (0, 0)
  line L5 (1.416111, 0) -> (0, 0)
  line L6 (0, 0) -> (0, 2.216498)
  point P0 (-16, 5)
  constraints: 8 end point, 2 perpendicular, 1 collinear, 1 horizontal, 1 point on line
sketch "Boceto71" plane through (17.416111, 1.000274, -4.5) normal (0.0013158, 0.9999991, 0) x (0.9999991, -0.0013158, 0)
  line L0 (-18.791765, 0) -> (-18.791617, -0.25)
  line L1 (-18.791765, 1) -> (0, 1)
  line L2 (-18.791765, 0) -> (0, 1)
  line L3 (0.208219, 0) -> (-18.791765, 0)
  line L4 (0, 0) -> (0, 1)
  line L5 (0, 0.49264) -> (0.002064, 0.491349)
  line L6 (0.002064, 0.491349) -> (-18.791765, 0.576357)
  line L7 (-18.791765, 1) -> (-18.791765, 0.576357)
  line L8 (-18.791765, -0.25) -> (0.208252, -0.25)
  point P0 (-17.41478, -4.5)
  constraints: 8 end point, 1 perpendicular, 1 point on line
sketch "Boceto71 outline for Extrusión56" plane through (17.416111, 1.000274, -4.5) normal (0.0013158, 0.9999991, 0) x (0.9999991, -0.0013158, 0)
  line L0 (0, 1) -> (-18.791765, 1)
  line L1 (0, 0.49264) -> (0, 1)
  line L2 (-18.791765, 0.576357) -> (-0.000006, 0.491358)
  line L3 (-18.791765, 1) -> (-18.791765, 0.576357)
extrude "Extrusión56" add sketch "Boceto71 outline for Extrusión56" along normal blind 0.3
sketch "Boceto72" plane through (0, 0, -5) normal (0, 0, -1) x (-1, 0, 0)
  line L0 (-17.624362, 0) -> (1.376954, 0.025002)
  line L1 (-17.624362, 0) -> (-17.624362, -1.002119)
  line L2 (-17.624362, -1.002119) -> (0, -1.002119)
  line L3 (0, -12) -> (0, 0)
  line L4 (0, -1.002119) -> (0, 0)
  line L5 (-16, 0) -> (-16, -12)
  line L6 (0, 0) -> (-16, 0)
  line L7 (-17.624362, -1.002119) -> (-17.624362, 0)
  line L8 (0, 0) -> (0, -1.002119)
  line L9 (0, -1.002119) -> (-17.624362, -1.002119)
  line L10 (-17.624362, -1.002119) -> (-17.624362, 0)
  line L11 (0, 0) -> (-16, 0)
  line L12 (-17.624362, 0) -> (0, 0)
  constraints: 18 end point, 3 collinear, 3 perpendicular, 1 horizontal, 1 parallel, 1 point on line, 1 vertical
extrude "Extrusión57" add sketch "Boceto72" along normal blind 0.5
sketch "Boceto73" plane through (0, -1.002119, -5) normal (-1, 0, 0) x (0, 0, 1)
  line L0 (0, -10.997881) -> (0, 0)
  line L1 (0, 0) -> (-0.5, 0)
  line L2 (-0.5, 0) -> (-0.5, 1.002119)
  line L3 (-0.5, 1.002119) -> (0, 1.002119)
  line L4 (0, 1.002119) -> (0, 0)
  point P0 (5, 1.002119)
  constraints: 8 end point, 2 parallel, 1 horizontal, 1 perpendicular
extrude "Extrusión58" add sketch "Boceto73" along normal blind 1.35
sketch "Boceto74" plane through (16, 0, -5) normal (0, -1, 0) x (1, 0, 0)
  line L0 (1.416111, 0) -> (1.416111, -0.5)
  line L1 (1.416111, -0.5) -> (1.416111, 0.5)
  line L2 (1.416111, 0.5) -> (0, 2.216498)
  line L3 (1.416111, 0.5) -> (0, 2.216498)
  line L4 (0, 2.216498) -> (0, 0)
  line L5 (0, 0) -> (1.416111, -0.5)
  point P0 (-16, 5)
  constraints: 8 end point, 1 collinear, 1 parallel, 1 vertical
extrude "Extrusión59" add sketch "Boceto74" along normal blind 12.5
